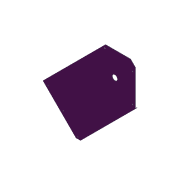
# Autodesk Inventor part: Shooter Plate
Saved by Autodesk Inventor 2012 (Build 160160000, 160)
## iProperties
Created: 2013-01-15
Part Number: Shooter Plate
Material: Aluminum-6061
Document SubType Name: Modeling
Designer: William
Density: 2.71 g/cm^3
Mass: 605.461 g
Surface Area: 2840.38 cm^2
Volume: 223.417 cm^3
Author: William
Autodesk Inventor part; units mm, degrees
note: some values were not read from the file. Chosen so that the rebuilt part matches the saved one: second side of "Extrusion16".
ref_plane "YZ Plane" through (0, 0, 0) normal (1, 0, 0) x (0, 1, 0)
ref_plane "XZ Plane" through (0, 0, 0) normal (0, 1, 0) x (-1, 0, 0)
ref_plane "XY Plane" through (0, 0, 0) normal (0, 0, 1) x (1, 0, 0)
sketch "Sketch1" plane through (0, 0, 0) normal (0, 0, 1) x (1, 0, 0)
  line L0 (220.8897, 190.2129) -> (246.2897, 164.8129)
  line L1 (246.2897, 164.8129) -> (246.2897, -38.3871)
  line L2 (246.2897, -38.3871) -> (-33.1103, -317.7871)
  line L3 (-102.9603, -317.7871) -> (-261.7103, -159.0371)
  line L4 (-261.7103, -159.0371) -> (87.5397, 190.2129)
  circle A0 centre (233.5897, -12.9871) radius 3.175
  circle A1 centre (233.5897, 139.4129) radius 3.175
  circle A2 centre (84.9068, 172.8665) radius 3.175
  line L5 (84.9068, 172.8665) -> (233.5897, 139.4129) construction
  line L6 (233.5897, 139.4129) -> (233.5897, -12.9871) construction
  line L7 (-102.9603, -317.7871) -> (-33.1103, -317.7871)
  circle A3 centre (138.3397, 63.2129) radius 14.2875
  line L8 (84.9068, 172.8665) -> (138.3397, 63.2129) construction
  line L9 (138.3397, 63.2129) -> (233.5897, 139.4129) construction
  line L10 (138.3397, 63.2129) -> (233.5897, -12.9871) construction
  circle A4 centre (-59.055, -307.8109) radius 3.175
  circle A5 centre (-216.809, -150.0569) radius 3.175
  circle A6 centre (-137.932, -228.9339) radius 3.175
  line L11 (87.5397, 190.2129) -> (220.8897, 190.2129)
  line L12 (-216.809, -150.0569) -> (-137.932, -228.9339) construction
  line L13 (-137.932, -228.9339) -> (-59.055, -307.8109) construction
  point P0 (0, 0)
  dimension "d222" = 203.2
  dimension "d228" = 12.7
  dimension "d229" = 152.4
  dimension "d230" = 25.4
  dimension "d233" = 135
  dimension "d236" = 6.35
  dimension "d237" = 381
  dimension "d238" = 107.95
  dimension "d240" = 508
  dimension "d241" = 158.75
  dimension "d242" = 28.575
  dimension "d247" = 279.4
  dimension "d248" = 508
  dimension "d249" = 6.35
  dimension "d250" = 38.1
  dimension "d252" = 25.4
  dimension "d253" = 25.4
  constraints: 28 end point, 7 centre point, 4 equal radius, 3 equal length, 3 perpendicular, 2 horizontal, 2 vertical, 1 collinear, 1 parallel, 1 other
  measures "d222" distance of L0.end L1.end
  measures "d228" distance between parallel lines of L1 L6
  measures "d229" distance of L5.end L6.end
  measures "d230" vertical distance of L1.end L6.end
  measures "d233" angle of L1 L0
  measures "d236" diameter of A2
  measures "d237" distance from line of L7 L8.end
  measures "d238" distance from line of L1 L8.end
  measures "d240" distance from line of L1 L3.end
  measures "d241" distance from line of L7 L3.end
  measures "d242" diameter of A3
  measures "d247" distance from line of L7 L1.end
  measures "d248" distance between parallel lines of L7 L11
  measures "d249" diameter of A6
  measures "d250" distance between parallel lines of L3 L12
  measures "d252" distance from line of L4 L12.start
  measures "d253" distance from line of L2 L13.end
extrude "Extrusion14" add sketch "Sketch1" along normal blind 1.5875
sketch "Sketch12" plane through (0, 0, 1.5875) normal (0, 0, 1) x (1, 0, 0)
  line L0 (-33.1103, -317.7871) -> (-102.9603, -317.7871) projected
  line L1 (246.2897, -38.3871) -> (-33.1103, -317.7871) projected
  line L2 (246.2897, 164.8129) -> (246.2897, -38.3871) projected
  line L3 (220.8897, 190.2129) -> (246.2897, 164.8129) projected
  line L4 (-46.5806, -317.7871) -> (246.2897, -24.9168)
  line L5 (246.2897, -24.9168) -> (246.2897, -38.3871)
  line L6 (-33.1103, -317.7871) -> (246.2897, -38.3871)
  line L7 (-46.5806, -317.7871) -> (-33.1103, -317.7871)
  point P0 (0, 0)
  dimension "d254" = 9.525
  constraints: 8 end point, 2 point on line, 1 horizontal, 1 parallel, 1 perpendicular, 1 vertical
  measures "d254" distance between parallel lines of L1 L4
extrude "Extrusion15" cut sketch "Sketch12" against normal up to next
sketch "Sketch13" plane through (0, 0, 1.5875) normal (0, 0, 1) x (1, 0, 0)
  line L0 (-46.5806, -317.7871) -> (246.2897, -24.9168) projected
  line L1 (-46.5806, -317.7871) -> (246.2897, -24.9168)
  line L2 (246.2897, -24.9168) -> (247.4123, -26.0393)
  line L3 (247.4123, -26.0393) -> (-45.4581, -318.9097)
  line L4 (-45.4581, -318.9097) -> (-46.5806, -317.7871)
  point P0 (0, 0)
  dimension "d257" = 1.5875
  constraints: 8 end point, 3 equal length, 1 perpendicular
  measures "d257" distance of L0.end L2.end
extrude "Extrusion16" add sketch "Sketch13" against normal blind 9.525
sketch "Sketch14" plane through (0, 0, 1.5875) normal (0, 0, 1) x (1, 0, 0)
  line L0 (-261.7103, -159.0371) -> (87.5397, 190.2129) projected
  line L1 (-102.9603, -317.7871) -> (-261.7103, -159.0371) projected
  line L2 (-46.5806, -317.7871) -> (-102.9603, -317.7871) projected
  line L3 (-261.7103, -159.0371) -> (-243.7497, -141.0766)
  line L4 (-243.7497, -141.0766) -> (-67.0392, -317.7871)
  line L5 (-67.0392, -317.7871) -> (-84.9997, -335.7476)
  line L6 (-84.9997, -335.7476) -> (-261.7103, -159.0371)
  point P0 (0, 0)
  dimension "d262" = 25.4
  constraints: 8 end point, 2 parallel, 2 point on line, 1 perpendicular
  measures "d262" distance of L4.end L5.end
extrude "Extrusion17" cut sketch "Sketch14" against normal up to next contours L0 L4 L2 L1
sketch "Sketch15" plane through (0, 0, 1.5875) normal (0, 0, 1) x (1, 0, 0)
  line L0 (-243.7497, -141.0766) -> (-67.0392, -317.7871) projected
  line L1 (-243.7497, -141.0766) -> (-67.0392, -317.7871)
  line L2 (-67.0392, -317.7871) -> (-68.1618, -318.9097)
  line L3 (-68.1618, -318.9097) -> (-244.8723, -142.1992)
  line L4 (-244.8723, -142.1992) -> (-243.7497, -141.0766)
  point P0 (0, 0)
  dimension "d266" = 1.5875
  constraints: 8 end point, 3 equal length, 1 perpendicular
  measures "d266" distance of L0.end L2.end
extrude "Extrusion18" add sketch "Sketch15" against normal blind 9.525
fillet "Fillet1" radius 0.3969 4 edges at (-156.517, -230.5544, 1.5875) (99.8545, -171.3519, 0) (-155.3945, -229.4319, 0) (100.9771, -172.4745, 1.5875)
body "Solid4"
